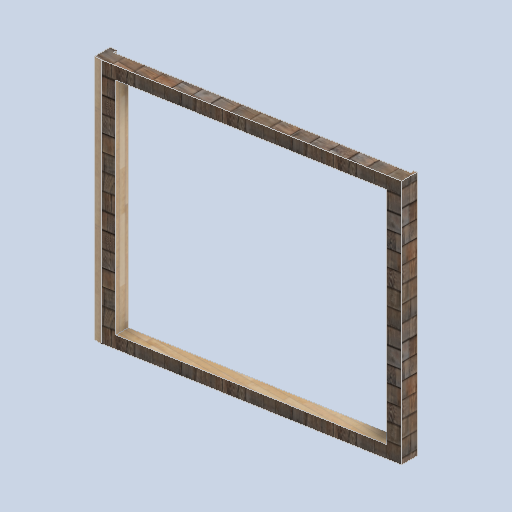
# Autodesk Inventor part: eave_frame_side_
Saved by Autodesk Inventor 2024.2 (Build 282272000, 272)
## iProperties
Created: 2024-05-23
Part Number: eave_frame_side_
Material: Wood (Maple)
Document SubType Name: Modeling
Designer: LOSTER_1
Density: 0.67 g/cm^3
Appearance: Natural Maple - Glossy Dark Tint
Author: LOSTER_1
Autodesk Inventor part; units mm, degrees
sketch "Sketch1" plane through (0, 0, 0) normal (1, 0, 0) x (0, 1, 0)
  line L0 (-16025.4384, 1509.0974) -> (-16025.4384, 1358.9468)
  line L1 (-15853.0538, 1508.6791) -> (-16025.4384, 1508.6791)
  line L2 (-13852.385, -1490.9026) -> (-13852.385, 1509.0974)
  line L3 (-13502.385, 1508.6791) -> (-13502.385, 1509.0974)
  line L4 (-13852.385, 1509.0974) -> (-13677.385, 1509.0974)
  line L5 (-15853.0538, -1491.3209) -> (-15853.0538, 1508.6791)
  line L6 (-16025.4384, 1358.9468) -> (-16025.4384, -1491.3209)
  line L7 (-16025.4384, -1491.3209) -> (-13677.385, -1491.3209)
  line L8 (-13677.385, -1491.3209) -> (-13677.385, 1509.0974)
  line L9 (-13677.385, 1508.6791) -> (-16025.4384, 1508.6791)
  line L10 (-16025.4384, 1508.6791) -> (-16025.4384, 1358.6791)
  line L11 (-16025.4384, 1508.6791) -> (-13677.385, 1508.6791)
  line L12 (-13677.385, 1508.6791) -> (-13677.385, 1358.6791)
  line L13 (-13677.385, 1358.6791) -> (-16025.4384, 1358.6791)
  line L14 (-16025.4384, 1358.6791) -> (-16025.4384, 1508.6791)
  point P0 (0, 0)
  dimension "d2" = 150
  constraints: 30 end point, 4 point on line, 3 perpendicular, 2 parallel, 1 coincident, 1 horizontal, 1 vertical
  measures "d2" distance of L1.end L10.end
ref_plane "Work Plane2" through (2500, 0, 0) normal (1, 0, 0) x (0, 1, 0)
ref_plane "Work Plane1" through (0, 0, 0) normal (1, 0, 0) x (0, 1, 0)
extrude "Extrusion1" add sketch "Sketch1" along normal blind 60 contours L1 L5 L13 L6 L0 | L9 L2 L13 L5 | L9 L8 L13 L2
ref_plane "Work Plane3" through (60, 0, 0) normal (1, 0, 0) x (0, 0, -1)
sketch "Sketch3" plane through (60, 0, 0) normal (1, 0, 0) x (0, 0, -1)
  line L0 (-1358.6791, -13677.385) -> (-1508.6791, -13677.385) projected
  line L1 (-1508.6791, -13677.385) -> (-1508.6791, -16025.4384) projected
  line L2 (-1508.6791, -16025.4384) -> (-1358.6791, -16025.4384) projected
  line L3 (-1358.6791, -16025.4384) -> (-1358.6791, -13677.385) projected
  point P0 (0, 0)
sketch "Sketch5" plane through (2500, 0, 0) normal (1, 0, 0) x (0, 1, 0)
  line L0 (-16025.4384, 1358.9468) -> (-16025.4384, -1491.3209) projected
  point P0 (0, 0)
ref_plane "Work Plane4" through (60, -16025.4384, 1508.6791) normal (0, -1, 0) x (0, 0, -1)
sketch "Sketch6" plane through (60, -16025.4384, 1508.6791) normal (0, -1, 0) x (0, 0, -1)
  line L0 (0, 0) -> (150, 0) projected
  line L1 (149.7323, 2440) -> (3000, 2440) projected
  line L2 (0, 0) -> (430.2378, 2440)
  line L3 (0, 0) -> (2477.6409, 0) construction
  line L4 (150, 0) -> (580.2378, 2440)
  line L5 (150, 0) -> (2627.6409, 0) construction
  line L6 (580.2378, 2440) -> (430.2378, 2440)
  point P0 (1508.6791, -60)
  dimension "d6" = 80
  dimension "d7" = 80
  constraints: 10 end point, 3 horizontal, 2 equal length, 2 point on line
  measures "d6" angle of L3 L2
  measures "d7" angle of L5 L4
sketch "Sketch9" plane through (2500, 0, 0) normal (1, 0, 0) x (0, 1, 0)
  line L0 (-13677.385, -1491.3209) -> (-13677.385, 1509.0974) projected
  line L1 (-16025.4384, 1078.4413) -> (-13677.385, 1078.4413)
  line L2 (-13677.385, 1078.4413) -> (-13677.385, 928.4413)
  line L3 (-13677.385, 928.4413) -> (-16025.4384, 928.4413)
  line L4 (-16025.4384, 928.4413) -> (-16025.4384, 1078.4413)
  point P0 (0, 0)
  point P1 (-16025.4384, 928.4413)
  constraints: 8 end point, 2 parallel, 1 horizontal, 1 perpendicular, 1 point on line
loft "Loft2" add profiles "Sketch9" section 2 edges at (60, -13677.385, 1433.6791) (60, -15939.2461, 1508.6791) (60, -16025.4384, 1433.813) (60, -14851.4117, 1358.6791)
sketch "Sketch10" plane through (0, -13677.385, 1508.6791) normal (0, 1, 0) x (1, 0, 0)
  line L0 (60, 150) -> (60, 120)
  line L1 (60, 120) -> (2472.779, 545.438)
  line L2 (60, 120) -> (2510, 120) construction
  line L3 (0, 150) -> (60, 150) projected
  line L4 (60, 150) -> (2472.779, 575.438)
  line L5 (2472.779, 545.438) -> (2472.779, 575.438)
  point P0 (0, 1508.6791)
  dimension "d16" = 30
  dimension "d17" = 2450
  dimension "d18" = 10
  dimension "d19" = 2450
  constraints: 10 end point, 2 vertical, 1 equal length, 1 horizontal
  measures "d16" distance of L0.start L0.end
  measures "d17" distance of L0.end L1.end
  measures "d18" angle of L2 L1
  measures "d19" distance of L0.start L4.end
extrude "Extrusion2" cut sketch "Sketch10" against normal through all
sketch "Sketch11" plane through (0, -16025.4384, 1508.6791) normal (0, 0, 1) x (1, 0, 0)
  line L0 (2500, 0) -> (2500, 2348.0534) projected
  line L1 (2500, 2348.0534) -> (60, 2348.0534) projected
  line L2 (60, 2348.0534) -> (60, 0) projected
  line L3 (2500, 0) -> (60, 0) projected
  line L4 (2500, 0) -> (60, 0) projected
  line L5 (2500, 0) -> (2380, 0)
  line L6 (2380, 0) -> (2380, 120)
  line L7 (2380, 120) -> (2500, 120)
  line L8 (2500, 120) -> (2500, 0)
  line L9 (60, 2348.0534) -> (180, 2348.0534)
  line L10 (180, 2348.0534) -> (180, 2228.0534)
  line L11 (180, 2228.0534) -> (60, 2228.0534)
  line L12 (60, 2228.0534) -> (60, 2348.0534)
  line L13 (2380, 120) -> (180, 120)
  line L14 (180, 120) -> (180, 2228.0534)
  line L15 (180, 2228.0534) -> (2380, 2228.0534)
  line L16 (2380, 2228.0534) -> (2380, 120)
  point P0 (0, 16025.4384)
  dimension "d22" = 120
  dimension "d23" = 120
  dimension "d24" = 120
  dimension "d25" = 120
  constraints: 24 end point, 6 parallel, 3 horizontal, 3 perpendicular
  measures "d22" distance of L6.end L7.end
  measures "d23" distance of L5.end L6.end
  measures "d24" distance of L10.end L11.end
  measures "d25" distance of L9.end L10.end
extrude "Extrusion3" cut sketch "Sketch11" against normal through all contours L13 L14 L15 L16
body "Solid1"
